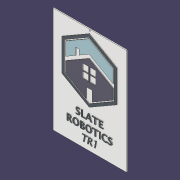
# Autodesk Inventor part: BP002b
Saved by Autodesk Inventor 2017 SP1 (Build 210196100, 196)
## iProperties
Created: 2017-12-18
Part Number: BP002b
Material: ABS Plastic
Document SubType Name: Modeling
Designer: Zach
Density: 1.06 g/cm^3
Appearance: CR White
Author: Zach
Autodesk Inventor part; units mm, degrees
ref_plane "YZ Plane" through (0, 0, 0) normal (1, 0, 0) x (0, 1, 0)
ref_plane "XZ Plane" through (0, 0, 0) normal (0, 1, 0) x (-1, 0, 0)
ref_plane "XY Plane" through (0, 0, 0) normal (0, 0, 1) x (1, 0, 0)
sketch "Sketch1" plane through (0, 0, 0) normal (0, 0, 1) x (1, 0, 0)
  line L0 (0, 0) -> (288, 0)
  line L1 (288, 0) -> (288, 415)
  line L2 (288, 415) -> (0, 415)
  line L3 (0, 415) -> (0, 0)
  line L4 (5, 5) -> (283, 5) construction
  line L5 (283, 5) -> (283, 410) construction
  line L6 (283, 410) -> (5, 410) construction
  line L7 (5, 410) -> (5, 5) construction
  circle A0 centre (5, 410) radius 2.5
  circle A1 centre (283, 410) radius 2.5
  circle A2 centre (283, 5) radius 2.5
  circle A3 centre (5, 5) radius 2.5
  dimension "d0" = 288
  dimension "d1" = 415
  dimension "d2" = 5
  dimension "d3" = 5
  dimension "d4" = 5
  dimension "d5" = 5
  dimension "d6" = 5
  constraints: 16 end point, 4 centre point, 4 coincident, 4 parallel, 2 perpendicular, 1 horizontal, 3 other
  measures "d0" distance of L2.end L1.end
  measures "d1" distance of L1.end L0.end
  measures "d2" distance between parallel lines of L3 L7
  measures "d3" diameter of A0
  measures "d4" diameter of A1
  measures "d5" diameter of A2
  measures "d6" diameter of A3
extrude "Extrusion1" add sketch "Sketch1" along normal blind 4 contours L3 L2 L1 L0 | A0 | A1 | A2 | A3
sketch "Sketch2" plane through (0, 0, 4) normal (0, 0, 1) x (1, 0, 0)
  line L0 (0, 150) -> (288, 150) construction
  line L1 (288, 150) -> (288, 0) construction
  line L2 (288, 0) -> (0, 0) construction
  line L3 (0, 0) -> (0, 150) construction
  line L4 (19, 400) -> (269, 400) construction
  line L5 (269, 400) -> (269, 150) construction
  line L6 (269, 150) -> (19, 150) construction
  line L7 (19, 150) -> (19, 400) construction
  line L8 (288, 415) -> (0, 415) projected
  line L9 (288, 0) -> (288, 415) projected
  line L10 (144, 400) -> (252.2532, 337.5)
  line L11 (252.2532, 337.5) -> (252.2532, 212.5)
  line L12 (252.2532, 212.5) -> (144, 150)
  line L13 (144, 150) -> (35.7468, 212.5)
  line L14 (35.7468, 212.5) -> (35.7468, 337.5)
  line L15 (35.7468, 337.5) -> (144, 400)
  line L16 (144, 388.2221) -> (242.0532, 331.611)
  line L17 (242.0532, 331.611) -> (242.0532, 218.389)
  line L18 (242.0532, 218.389) -> (144, 161.7779)
  line L19 (144, 161.7779) -> (45.9468, 218.389)
  line L20 (45.9468, 218.389) -> (45.9468, 331.611)
  line L21 (45.9468, 331.611) -> (144, 388.2221)
  line L22 (144, 383.3146) -> (237.8032, 329.1573) construction
  line L23 (237.8032, 329.1573) -> (237.8032, 220.8427) construction
  line L24 (237.8032, 220.8427) -> (144, 166.6854) construction
  line L25 (144, 166.6854) -> (50.1968, 220.8427) construction
  line L26 (50.1968, 220.8427) -> (50.1968, 329.1573) construction
  line L27 (50.1968, 329.1573) -> (144, 383.3146) construction
  line L28 (50.1968, 276.6573) -> (90.1968, 299.7513)
  line L29 (90.1968, 299.7513) -> (90.1968, 328.2513)
  line L30 (90.1968, 328.2513) -> (104.1968, 328.2513)
  line L31 (104.1968, 328.2513) -> (104.1968, 307.8342)
  line L32 (104.1968, 307.8342) -> (144, 330.8146)
  line L33 (144, 330.8146) -> (237.8032, 276.6573)
  line L34 (237.8032, 276.6573) -> (237.8032, 329.1573)
  line L35 (237.8032, 329.1573) -> (144, 383.3146)
  line L36 (144, 383.3146) -> (50.1968, 329.1573)
  line L37 (50.1968, 276.6573) -> (50.1968, 329.1573)
  line L38 (50.1968, 220.8427) -> (132, 173.6136)
  line L39 (132, 173.6136) -> (132, 213.6854)
  line L40 (132, 213.6854) -> (156, 213.6854)
  line L41 (156, 213.6854) -> (156, 173.6136)
  line L42 (156, 173.6136) -> (237.8032, 220.8427)
  line L43 (237.8032, 220.8427) -> (237.8032, 261.6573)
  line L44 (237.8032, 261.6573) -> (144, 315.8146)
  line L45 (144, 315.8146) -> (50.1968, 261.6573)
  line L46 (50.1968, 261.6573) -> (50.1968, 220.8427)
  line L47 (117.75, 287.6854) -> (170.25, 287.6854) construction
  line L48 (170.25, 287.6854) -> (170.25, 236.6854) construction
  line L49 (170.25, 236.6854) -> (117.75, 236.6854) construction
  line L50 (117.75, 236.6854) -> (117.75, 287.6854) construction
  line L51 (117.75, 236.6854) -> (141.75, 236.6854)
  line L52 (141.75, 236.6854) -> (141.75, 260.6854)
  line L53 (141.75, 260.6854) -> (117.75, 260.6854)
  line L54 (117.75, 260.6854) -> (117.75, 236.6854)
  line L55 (117.75, 287.6854) -> (141.75, 287.6854)
  line L56 (141.75, 287.6854) -> (141.75, 263.6854)
  line L57 (141.75, 263.6854) -> (117.75, 263.6854)
  line L58 (117.75, 263.6854) -> (117.75, 287.6854)
  line L59 (170.25, 287.6854) -> (146.25, 287.6854)
  line L60 (146.25, 287.6854) -> (146.25, 263.6854)
  line L61 (146.25, 263.6854) -> (170.25, 263.6854)
  line L62 (170.25, 263.6854) -> (170.25, 287.6854)
  line L63 (170.25, 236.6854) -> (146.25, 236.6854)
  line L64 (146.25, 236.6854) -> (146.25, 260.6854)
  line L65 (146.25, 260.6854) -> (170.25, 260.6854)
  line L66 (170.25, 260.6854) -> (170.25, 236.6854)
  line L67 (90.7483, 102.3958) -> (90.7483, 106.6804)
  spline S0 degree 2 poles (90.7483, 106.6804) (93.6748, 105.4563) (96.5631, 104.9781) (97.7682, 104.9781) knots 0 0 0 1 2 2 2
  spline S1 degree 2 poles (97.7682, 104.9781) (99.9487, 104.9781) (102.1102, 106.9291) (102.1102, 108.3063) knots 0 0 0 1 2 2 2
  spline S2 degree 2 poles (102.1102, 108.3063) (102.1102, 109.3583) (101.5172, 110.2) knots 0 0 0 1 1 1
  spline S3 degree 2 poles (101.5172, 110.2) (100.9051, 111.0224) (98.5524, 112.3423) knots 0 0 0 1 1 1
  line L68 (98.5524, 112.3423) -> (96.8692, 113.2795)
  spline S4 degree 2 poles (96.8692, 113.2795) (93.254, 115.2879) (91.9916, 116.9903) knots 0 0 0 1 1 1
  spline S5 degree 2 poles (91.9916, 116.9903) (90.6909, 118.6927) (90.6909, 120.9306) knots 0 0 0 1 1 1
  spline S6 degree 2 poles (90.6909, 120.9306) (90.6909, 123.7615) (95.0138, 127.7784) (99.0497, 127.7784) knots 0 0 0 1 2 2 2
  spline S7 degree 2 poles (99.0497, 127.7784) (102.0719, 127.7784) (105.8592, 126.9176) knots 0 0 0 1 1 1
  line L69 (105.8592, 126.9176) -> (105.8592, 122.9199)
  spline S8 degree 2 poles (105.8592, 122.9199) (101.9763, 124.3545) (99.7001, 124.3545) knots 0 0 0 1 1 1
  spline S9 degree 2 poles (99.7001, 124.3545) (97.8064, 124.3545) (95.8363, 122.7095) (95.8363, 121.5618) knots 0 0 0 1 2 2 2
  spline S10 degree 2 poles (95.8363, 121.5618) (95.8363, 120.682) (96.4484, 119.936) knots 0 0 0 1 1 1
  spline S11 degree 2 poles (96.4484, 119.936) (97.0222, 119.1709) (99.3749, 117.8511) knots 0 0 0 1 1 1
  line L70 (99.3749, 117.8511) -> (101.1729, 116.8564)
  spline S12 degree 2 poles (101.1729, 116.8564) (105.3236, 114.542) (106.4522, 112.8396) knots 0 0 0 1 1 1
  spline S13 degree 2 poles (106.4522, 112.8396) (107.5807, 111.1181) (107.5807, 108.9758) knots 0 0 0 1 1 1
  spline S14 degree 2 poles (107.5807, 108.9758) (107.5807, 105.8962) (102.8944, 101.5542) (97.7873, 101.5542) knots 0 0 0 1 2 2 2
  spline S15 degree 2 poles (97.7873, 101.5542) (94.7651, 101.5542) (90.7483, 102.3958) knots 0 0 0 1 1 1
  line L71 (111.9036, 102.1663) -> (111.9036, 127.1663)
  line L72 (111.9036, 127.1663) -> (117.1064, 127.1663)
  line L73 (117.1064, 127.1663) -> (117.1064, 105.7049)
  line L74 (117.1064, 105.7049) -> (128.2578, 105.7049)
  line L75 (128.2578, 105.7049) -> (128.2578, 102.1663)
  line L76 (128.2578, 102.1663) -> (111.9036, 102.1663)
  line L77 (129.2716, 102.1663) -> (138.9694, 127.1663)
  line L78 (138.9694, 127.1663) -> (144.1913, 127.1663)
  line L79 (144.1913, 127.1663) -> (153.9273, 102.1663)
  line L80 (153.9273, 102.1663) -> (148.5907, 102.1663)
  line L81 (148.5907, 102.1663) -> (145.9893, 108.8419)
  line L82 (145.9893, 108.8419) -> (135.6603, 108.8419)
  line L83 (135.6603, 108.8419) -> (133.0589, 102.1663)
  line L84 (133.0589, 102.1663) -> (129.2716, 102.1663)
  line L85 (136.9419, 112.1701) -> (144.6886, 112.1701)
  line L86 (144.6886, 112.1701) -> (140.8248, 122.1357)
  line L87 (140.8248, 122.1357) -> (136.9419, 112.1701)
  line L88 (163.6825, 102.1663) -> (163.6825, 123.7233)
  line L89 (163.6825, 123.7233) -> (154.7307, 123.7233)
  line L90 (154.7307, 123.7233) -> (154.7307, 127.1663)
  line L91 (154.7307, 127.1663) -> (177.837, 127.1663)
  line L92 (177.837, 127.1663) -> (177.837, 123.7233)
  line L93 (177.837, 123.7233) -> (168.8852, 123.7233)
  line L94 (168.8852, 123.7233) -> (168.8852, 102.1663)
  line L95 (168.8852, 102.1663) -> (163.6825, 102.1663)
  line L96 (181.3183, 102.1663) -> (181.3183, 127.1663)
  line L97 (181.3183, 127.1663) -> (197.3282, 127.1663)
  line L98 (197.3282, 127.1663) -> (197.3282, 123.7233)
  line L99 (197.3282, 123.7233) -> (186.521, 123.7233)
  line L100 (186.521, 123.7233) -> (186.521, 116.7608)
  line L101 (186.521, 116.7608) -> (195.4537, 116.7608)
  line L102 (195.4537, 116.7608) -> (195.4537, 113.3178)
  line L103 (195.4537, 113.3178) -> (186.521, 113.3178)
  line L104 (186.521, 113.3178) -> (186.521, 105.7049)
  line L105 (186.521, 105.7049) -> (198.1316, 105.7049)
  line L106 (198.1316, 105.7049) -> (198.1316, 102.1663)
  line L107 (198.1316, 102.1663) -> (181.3183, 102.1663)
  line L108 (55.9836, 62.2098) -> (55.9836, 87.2098)
  line L109 (55.9836, 87.2098) -> (65.337, 87.2098)
  spline S16 degree 2 poles (65.337, 87.2098) (68.2062, 87.2098) (71.2093, 85.7752) (72.9499, 82.8486) (72.9499, 81.0124) knots 0 0 0 1 2 3 3 3
  spline S17 degree 2 poles (72.9499, 81.0124) (72.9499, 78.8127) (70.425, 74.9106) (68.1106, 73.8777) knots 0 0 0 1 2 2 2
  line L110 (68.1106, 73.8777) -> (76.2781, 62.2098)
  line L111 (76.2781, 62.2098) -> (69.9468, 62.2098)
  line L112 (69.9468, 62.2098) -> (63.7303, 72.424)
  line L113 (63.7303, 72.424) -> (60.8803, 72.424)
  line L114 (60.8803, 72.424) -> (60.8803, 62.2098)
  line L115 (60.8803, 62.2098) -> (55.9836, 62.2098)
  line L116 (60.8803, 75.8479) -> (62.0662, 75.8479)
  spline S18 degree 2 poles (62.0662, 75.8479) (65.2797, 75.8479) (67.7471, 78.6597) (67.7471, 80.4385) knots 0 0 0 1 2 2 2
  spline S19 degree 2 poles (67.7471, 80.4385) (67.7471, 81.9688) (65.7578, 83.7859) (62.6974, 83.7859) knots 0 0 0 1 2 2 2
  line L117 (62.6974, 83.7859) -> (60.8803, 83.7859)
  line L118 (60.8803, 83.7859) -> (60.8803, 75.8479)
  spline S20 degree 2 poles (90.9683, 61.5977) (87.0662, 61.5977) (81.2896, 64.8303) (78.2865, 70.8747) (78.2865, 74.7193) knots 0 0 0 1 2 3 3 3
  spline S21 degree 2 poles (78.2865, 74.7193) (78.2865, 78.5258) (81.2896, 84.6084) (87.1044, 87.8219) (90.9683, 87.8219) knots 0 0 0 1 2 3 3 3
  spline S22 degree 2 poles (90.9683, 87.8219) (94.8129, 87.8219) (100.6278, 84.6084) (103.6308, 78.5258) (103.6308, 74.7193) knots 0 0 0 1 2 3 3 3
  spline S23 degree 2 poles (103.6308, 74.7193) (103.6308, 70.8747) (100.6278, 64.8303) (94.8703, 61.5977) (90.9683, 61.5977) knots 0 0 0 1 2 3 3 3
  spline S24 degree 2 poles (90.9683, 65.0216) (94.5834, 65.0216) (98.1029, 70.9129) (98.1029, 74.7193) knots 0 0 0 1 2 2 2
  spline S25 degree 2 poles (98.1029, 74.7193) (98.1029, 78.5449) (94.5643, 84.398) (90.9683, 84.398) knots 0 0 0 1 2 2 2
  spline S26 degree 2 poles (90.9683, 84.398) (87.3531, 84.398) (83.8145, 78.5449) (83.8145, 74.7193) knots 0 0 0 1 2 2 2
  spline S27 degree 2 poles (83.8145, 74.7193) (83.8145, 70.9129) (87.334, 65.0216) (90.9683, 65.0216) knots 0 0 0 1 2 2 2
  line L119 (108.298, 62.2098) -> (108.298, 87.2098)
  line L120 (108.298, 87.2098) -> (116.7334, 87.2098)
  spline S28 degree 2 poles (116.7334, 87.2098) (119.7938, 87.2098) (122.7204, 85.8326) (124.3845, 83.1547) (124.3845, 81.6436) knots 0 0 0 1 2 3 3 3
  spline S29 degree 2 poles (124.3845, 81.6436) (124.3845, 79.7691) (121.7831, 76.3261) (118.4166, 75.274) knots 0 0 0 1 2 2 2
  spline S30 degree 2 poles (118.4166, 75.274) (121.0945, 74.6046) (123.9254, 72.6535) (125.3982, 69.9374) (125.3982, 68.388) knots 0 0 0 1 2 3 3 3
  spline S31 degree 2 poles (125.3982, 68.388) (125.3982, 66.7048) (123.6767, 63.7783) (120.6546, 62.2098) (117.5176, 62.2098) knots 0 0 0 1 2 3 3 3
  line L121 (117.5176, 62.2098) -> (108.298, 62.2098)
  line L122 (113.2904, 65.7484) -> (114.285, 65.7484)
  spline S32 degree 2 poles (114.285, 65.7484) (117.0012, 65.7484) (118.9713, 66.4561) (119.966, 68.0437) (119.966, 69.0193) knots 0 0 0 1 2 3 3 3
  spline S33 degree 2 poles (119.966, 69.0193) (119.966, 70.8747) (116.6951, 73.4569) (114.1894, 73.4569) knots 0 0 0 1 2 2 2
  line L123 (114.1894, 73.4569) -> (113.2904, 73.4569)
  line L124 (113.2904, 73.4569) -> (113.2904, 65.7484)
  line L125 (113.2904, 76.8043) -> (114.3998, 76.8043)
  spline S34 degree 2 poles (114.3998, 76.8043) (116.7716, 76.8043) (119.1052, 79.157) (119.1052, 80.8402) knots 0 0 0 1 2 2 2
  spline S35 degree 2 poles (119.1052, 80.8402) (119.1052, 81.7392) (118.4166, 83.0591) (116.676, 83.7859) (114.2276, 83.7859) knots 0 0 0 1 2 3 3 3
  line L126 (114.2276, 83.7859) -> (113.2904, 83.7859)
  line L127 (113.2904, 83.7859) -> (113.2904, 76.8043)
  spline S36 degree 2 poles (141.2169, 61.5977) (137.3148, 61.5977) (131.5383, 64.8303) (128.5352, 70.8747) (128.5352, 74.7193) knots 0 0 0 1 2 3 3 3
  spline S37 degree 2 poles (128.5352, 74.7193) (128.5352, 78.5258) (131.5383, 84.6084) (137.3531, 87.8219) (141.2169, 87.8219) knots 0 0 0 1 2 3 3 3
  spline S38 degree 2 poles (141.2169, 87.8219) (145.0616, 87.8219) (150.8764, 84.6084) (153.8795, 78.5258) (153.8795, 74.7193) knots 0 0 0 1 2 3 3 3
  spline S39 degree 2 poles (153.8795, 74.7193) (153.8795, 70.8747) (150.8764, 64.8303) (145.119, 61.5977) (141.2169, 61.5977) knots 0 0 0 1 2 3 3 3
  spline S40 degree 2 poles (141.2169, 65.0216) (144.8321, 65.0216) (148.3516, 70.9129) (148.3516, 74.7193) knots 0 0 0 1 2 2 2
  spline S41 degree 2 poles (148.3516, 74.7193) (148.3516, 78.5449) (144.8129, 84.398) (141.2169, 84.398) knots 0 0 0 1 2 2 2
  spline S42 degree 2 poles (141.2169, 84.398) (137.6018, 84.398) (134.0631, 78.5449) (134.0631, 74.7193) knots 0 0 0 1 2 2 2
  spline S43 degree 2 poles (134.0631, 74.7193) (134.0631, 70.9129) (137.5826, 65.0216) (141.2169, 65.0216) knots 0 0 0 1 2 2 2
  line L128 (164.7632, 62.2098) -> (164.7632, 83.7668)
  line L129 (164.7632, 83.7668) -> (155.8114, 83.7668)
  line L130 (155.8114, 83.7668) -> (155.8114, 87.2098)
  line L131 (155.8114, 87.2098) -> (178.9178, 87.2098)
  line L132 (178.9178, 87.2098) -> (178.9178, 83.7668)
  line L133 (178.9178, 83.7668) -> (169.966, 83.7668)
  line L134 (169.966, 83.7668) -> (169.966, 62.2098)
  line L135 (169.966, 62.2098) -> (164.7632, 62.2098)
  line L136 (182.399, 62.2098) -> (182.399, 87.2098)
  line L137 (182.399, 87.2098) -> (187.6018, 87.2098)
  line L138 (187.6018, 87.2098) -> (187.6018, 62.2098)
  line L139 (187.6018, 62.2098) -> (182.399, 62.2098)
  spline S44 degree 2 poles (213.979, 63.2044) (212.334, 62.4776) (209.9047, 61.942) (206.8252, 61.5977) (205.3141, 61.5977) knots 0 0 0 1 2 3 3 3
  spline S45 degree 2 poles (205.3141, 61.5977) (198.7533, 61.5977) (192.3072, 68.981) (192.3072, 74.7193) knots 0 0 0 1 2 2 2
  spline S46 degree 2 poles (192.3072, 74.7193) (192.3072, 80.4577) (198.7341, 87.8219) (205.6393, 87.8219) knots 0 0 0 1 2 2 2
  spline S47 degree 2 poles (205.6393, 87.8219) (209.7135, 87.8219) (213.7494, 86.8655) knots 0 0 0 1 1 1
  line L140 (213.7494, 86.8655) -> (213.7494, 82.7913)
  spline S48 degree 2 poles (213.7494, 82.7913) (211.7984, 83.4607) (209.3309, 84.092) (207.1312, 84.398) (206.0218, 84.398) knots 0 0 0 1 2 3 3 3
  spline S49 degree 2 poles (206.0218, 84.398) (201.7181, 84.398) (197.8351, 78.8701) (197.8351, 74.7767) knots 0 0 0 1 2 2 2
  spline S50 degree 2 poles (197.8351, 74.7767) (197.8351, 70.4921) (202.2345, 65.1937) (206.5956, 65.1937) knots 0 0 0 1 2 2 2
  spline S51 degree 2 poles (206.5956, 65.1937) (210.2299, 65.1937) (213.979, 67.03) knots 0 0 0 1 1 1
  line L141 (213.979, 67.03) -> (213.979, 63.2044)
  line L142 (217.0968, 62.4393) -> (217.0968, 66.7239)
  spline S52 degree 2 poles (217.0968, 66.7239) (220.0233, 65.4998) (222.9116, 65.0216) (224.1167, 65.0216) knots 0 0 0 1 2 2 2
  spline S53 degree 2 poles (224.1167, 65.0216) (226.2973, 65.0216) (228.4587, 66.9726) (228.4587, 68.3498) knots 0 0 0 1 2 2 2
  spline S54 degree 2 poles (228.4587, 68.3498) (228.4587, 69.4018) (227.8657, 70.2434) knots 0 0 0 1 1 1
  spline S55 degree 2 poles (227.8657, 70.2434) (227.2536, 71.0659) (224.9009, 72.3858) knots 0 0 0 1 1 1
  line L143 (224.9009, 72.3858) -> (223.2177, 73.323)
  spline S56 degree 2 poles (223.2177, 73.323) (219.6025, 75.3314) (218.3401, 77.0338) knots 0 0 0 1 1 1
  spline S57 degree 2 poles (218.3401, 77.0338) (217.0394, 78.7362) (217.0394, 80.9741) knots 0 0 0 1 1 1
  spline S58 degree 2 poles (217.0394, 80.9741) (217.0394, 83.805) (221.3623, 87.8219) (225.3982, 87.8219) knots 0 0 0 1 2 2 2
  spline S59 degree 2 poles (225.3982, 87.8219) (228.4204, 87.8219) (232.2077, 86.9611) knots 0 0 0 1 1 1
  line L144 (232.2077, 86.9611) -> (232.2077, 82.9634)
  spline S60 degree 2 poles (232.2077, 82.9634) (228.3248, 84.398) (226.0486, 84.398) knots 0 0 0 1 1 1
  spline S61 degree 2 poles (226.0486, 84.398) (224.1549, 84.398) (222.1848, 82.753) (222.1848, 81.6053) knots 0 0 0 1 2 2 2
  spline S62 degree 2 poles (222.1848, 81.6053) (222.1848, 80.7255) (222.7969, 79.9795) knots 0 0 0 1 1 1
  spline S63 degree 2 poles (222.7969, 79.9795) (223.3707, 79.2144) (225.7234, 77.8946) knots 0 0 0 1 1 1
  line L145 (225.7234, 77.8946) -> (227.5214, 76.8999)
  spline S64 degree 2 poles (227.5214, 76.8999) (231.6722, 74.5854) (232.8007, 72.8831) knots 0 0 0 1 1 1
  spline S65 degree 2 poles (232.8007, 72.8831) (233.9292, 71.1616) (233.9292, 69.0193) knots 0 0 0 1 1 1
  spline S66 degree 2 poles (233.9292, 69.0193) (233.9292, 65.9397) (229.2429, 61.5977) (224.1358, 61.5977) knots 0 0 0 1 2 2 2
  spline S67 degree 2 poles (224.1358, 61.5977) (221.1136, 61.5977) (217.0968, 62.4393) knots 0 0 0 1 1 1
  line L146 (120.3462, 22.2216) -> (124.8077, 44.5678)
  line L147 (124.8077, 44.5678) -> (115.9231, 44.5678)
  line L148 (115.9231, 44.5678) -> (116.4423, 47.2216)
  line L149 (116.4423, 47.2216) -> (137.7308, 47.2216)
  line L150 (137.7308, 47.2216) -> (137.1923, 44.5678)
  line L151 (137.1923, 44.5678) -> (128.3269, 44.5678)
  line L152 (128.3269, 44.5678) -> (123.8846, 22.2216)
  line L153 (123.8846, 22.2216) -> (120.3462, 22.2216)
  line L154 (136.1346, 22.2216) -> (141.1154, 47.2216)
  line L155 (141.1154, 47.2216) -> (148.6538, 47.2216)
  spline S68 degree 2 poles (148.6538, 47.2216) (150.6346, 47.2216) (153.3462, 46.5485) (155.1346, 44.1255) (155.1346, 42.3755) knots 0 0 0 1 2 3 3 3
  spline S69 degree 2 poles (155.1346, 42.3755) (155.1346, 39.837) (151.5192, 35.337) (148.4423, 34.1639) knots 0 0 0 1 2 2 2
  line L156 (148.4423, 34.1639) -> (154.3846, 22.2216)
  line L157 (154.3846, 22.2216) -> (150.4615, 22.2216)
  line L158 (150.4615, 22.2216) -> (145.2115, 33.2793)
  line L159 (145.2115, 33.2793) -> (141.8654, 33.2793)
  line L160 (141.8654, 33.2793) -> (139.6731, 22.2216)
  line L161 (139.6731, 22.2216) -> (136.1346, 22.2216)
  line L162 (142.3846, 35.8947) -> (144.3462, 35.8947)
  spline S70 degree 2 poles (144.3462, 35.8947) (146.4423, 35.8947) (149.5385, 37.4716) (151.3654, 40.4716) (151.3654, 41.9716) knots 0 0 0 1 2 3 3 3
  spline S71 degree 2 poles (151.3654, 41.9716) (151.3654, 43.2601) (149.4038, 44.5678) (146.3654, 44.5678) knots 0 0 0 1 2 2 2
  line L163 (146.3654, 44.5678) -> (144.1154, 44.5678)
  line L164 (144.1154, 44.5678) -> (142.3846, 35.8947)
  line L165 (163.8269, 22.2216) -> (168.3077, 44.6832)
  line L166 (168.3077, 44.6832) -> (164.4038, 44.6832)
  line L167 (164.4038, 44.6832) -> (164.8269, 46.7601)
  line L168 (164.8269, 46.7601) -> (172.2115, 47.4332)
  line L169 (172.2115, 47.4332) -> (167.1538, 22.2216)
  line L170 (167.1538, 22.2216) -> (163.8269, 22.2216)
  point P0 (144, 275)
  point P1 (144, 213.6854)
  point P2 (144, 287.6854)
  dimension "d21" = 15
  dimension "d27" = 250
  dimension "d31" = 10.2
  dimension "d32" = 4.25
  dimension "d41" = 52.5
  dimension "d42" = 40
  dimension "d43" = 14
  dimension "d44" = 28.5
  dimension "d46" = 15
  dimension "d48" = 24
  dimension "d49" = 47
  dimension "d50" = 23
  dimension "d52" = 51
  dimension "d53" = 52.5
  dimension "d54" = 24
  dimension "d55" = 24
  dimension "d56" = 24
  dimension "d57" = 24
  dimension "d58" = 24
  dimension "d59" = 24
  dimension "d60" = 24
  dimension "d61" = 24
  constraints: 114 end point, 15 parallel, 9 perpendicular, 8 point on line, 5 horizontal, 5 midpoint, 5 vertical alignment, 4 collinear, 2 coincident, 2 vertical, 27 other
  measures "d21" distance between parallel lines of L8 L4
  measures "d27" distance of L4.start L4.end
  measures "d31" distance between parallel lines of L15 L21
  measures "d32" distance between parallel lines of L21 L27
  measures "d41" distance of L28.start L26.end
  measures "d42" distance between parallel lines of L26 L29
  measures "d43" distance of L29.end L30.end
  measures "d44" distance of L28.end L29.end
  measures "d46" distance of L32.end L44.end
  measures "d48" distance between parallel lines of L41 L39
  measures "d49" distance from line of L24.end L40
  measures "d50" distance between parallel lines of L40 L49
  measures "d52" distance of L49.end L47.start
  measures "d53" distance of L47.start L47.end
  measures "d54" distance of L53.end L52.end
  measures "d55" distance of L52.end L51.end
  measures "d56" distance of L56.end L57.end
  measures "d57" distance of L55.end L56.end
  measures "d58" distance of L61.end L60.end
  measures "d59" distance of L60.end L59.end
  measures "d60" distance of L64.end L65.end
  measures "d61" distance of L63.end L64.end
extrude "Extrusion2" add sketch "Sketch2" along normal blind 2
sketch "Sketch4" plane through (0, 0, 4) normal (0, 0, 1) x (1, 0, 0)
  line L0 (288, 415) -> (0, 415) projected
  circle A0 centre (144, 410) radius 2.5
  point P0 (0, 0)
  point P1 (144, 415)
  dimension "d63" = 5
  dimension "d64" = 5
  constraints: 1 centre point, 1 midpoint, 1 vertical alignment
  measures "d63" diameter of A0
  measures "d64" distance from line of L0 A0.centre
extrude "Extrusion3" cut sketch "Sketch4" against normal through all
body "Solid1"
